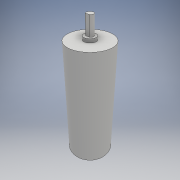
# Autodesk Inventor part: Motor
Saved by Autodesk Inventor 2018 (Build 220112000, 112)
## iProperties
Created: 2019-11-10
Part Number: Motor
Material: Типовые
Document SubType Name: Modeling
Designer: cosko
Density: 1 g/cm^3
Appearance: По умолчанию
Mass: 30.5037 g
Surface Area: 78.8452 cm^2
Volume: 30.5037 cm^3
Author: cosko
Autodesk Inventor part; units mm, degrees
ref_plane "YZ Plane" through (0, 0, 0) normal (1, 0, 0) x (0, 1, 0)
ref_plane "XZ Plane" through (0, 0, 0) normal (0, 1, 0) x (-1, 0, 0)
ref_plane "XY Plane" through (0, 0, 0) normal (0, 0, 1) x (1, 0, 0)
sketch "Эскиз2" plane through (0, 0, 0) normal (0, 0, 1) x (1, 0, 0)
  circle A0 centre (0, 0) radius 12.5
  circle A1 centre (0, 0) radius 3.5
  arc A2 (1.3229, -1.5) -> (-1.3229, -1.5) centre (0, 0) ccw
  line L0 (0, 2) -> (0, -1.5) construction
  line L1 (1.3229, -1.5) -> (-1.3229, -1.5)
  dimension "d2" = 25
  dimension "d3" = 7
  dimension "d4" = 4
  dimension "d5" = 3.5
  constraints: 4 end point, 3 centre point, 3 coincident, 3 point on circle, 1 horizontal, 1 vertical
  measures "d2" diameter of A0
  measures "d3" diameter of A1
  measures "d4" diameter of A2
  measures "d5" distance of L0.start L0.end
extrude "Выдавливание1" add sketch "Эскиз2" along normal blind 12 contours L1 A2
extrude "Выдавливание2" add sketch "Эскиз2" along normal blind 2 contours A1
extrude "Выдавливание3" add sketch "Эскиз2" against normal blind 67 contours A0
